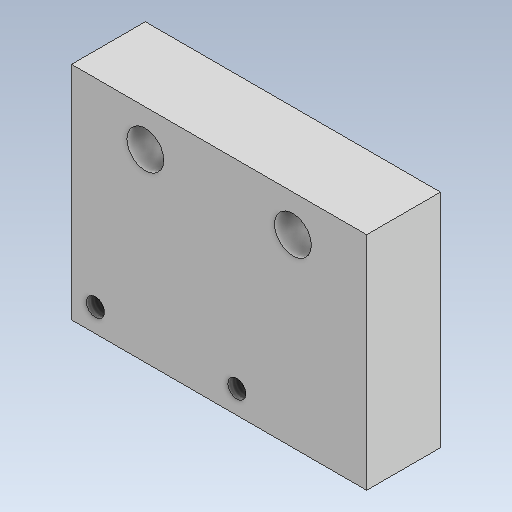
# Autodesk Inventor part: 0008-10-056
Saved by Autodesk Inventor 2020 (Build 240168000, 168)
## iProperties
Created: 2021-03-10
Part Number: 0008-10-056
Material: Generic
Document SubType Name: Modeling
Designer: Iulian Bors
Density: 1 g/cm^3
Appearance: Default
Description: Suport Senzor
Mass: 11.5123 g
Surface Area: 41.7113 cm^2
Volume: 11.5123 cm^3
Author: Iulian Bors
Subject: 056
Autodesk Inventor part; units mm, degrees
ref_plane "YZ Plane" through (0, 0, 0) normal (1, 0, 0) x (0, 1, 0)
ref_plane "XZ Plane" through (0, 0, 0) normal (0, 1, 0) x (-1, 0, 0)
ref_plane "XY Plane" through (0, 0, 0) normal (0, 0, 1) x (1, 0, 0)
sketch "Sketch1" plane through (0, 0, 0) normal (0, 0, 1) x (1, 0, 0)
  line L0 (-20, 15) -> (20, 15)
  line L1 (20, 15) -> (20, -15)
  line L2 (20, -15) -> (-20, -15)
  line L3 (-20, -15) -> (-20, 15)
  point P0 (0, 0)
  point P1 (0, 15)
  point P2 (-20, 0)
  dimension "d0" = 40
  dimension "d1" = 30
  constraints: 8 end point, 2 midpoint, 2 parallel, 1 horizontal, 1 horizontal alignment, 1 perpendicular, 1 vertical alignment
  measures "d0" distance of L0.start L0.end
  measures "d1" distance of L0.end L1.end
extrude "Extrusion1" add sketch "Sketch1" along normal blind 10
sketch "Sketch2" plane through (0, 0, 10) normal (0, 0, 1) x (1, 0, 0)
  line L0 (20, 15) -> (-20, 15) projected
  line L1 (20, -15) -> (20, 15) projected
  line L2 (-20, 15) -> (-20, -15) projected
  point P0 (0, 0)
  point P1 (10, 10)
  point P2 (-10, 10)
  dimension "d4" = 5
  dimension "d5" = 10
  dimension "d6" = 10
  constraints: 1 horizontal alignment
  measures "d4" distance from line of L0 point (10, 10)
  measures "d5" distance from line of point (10, 10) L1
  measures "d6" distance from line of L2 point (-10, 10)
hole "Hole1" at (10, 10, 10) at (-10, 10, 10) direction (0, 0, -1) diameter 5 end through all
sketch "Sketch3" plane through (0, 0, 10) normal (0, 0, 1) x (1, 0, 0)
  circle A0 centre (2.4125, -11.8725) radius 1.7875 projected
  circle A1 centre (-16.7625, -11.8725) radius 1.7875 projected
  point P0 (0, 0)
hole "Hole2" at (2.4125, -11.8725, 10) at (-16.7625, -11.8725, 10) direction (0, 0, -1) diameter 2.459 end through all thread size "M3x0.5" class "6H" standard "ISO Metric profile"
body "Solid1"
